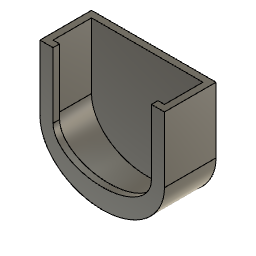
klarsteinHolder (Autodesk Fusion 360 design; units mm, degrees)
Autodesk Fusion 360 part; units mm, degrees
note: some values were not read from the file. Set by a fixed rule: which sketch regions a step uses.
sketch "out" plane through (0, 0, 0) normal (0, 1, 0) x (1, 0, 0)
  line L0 (0, 0) -> (57, 0)
  line L1 (57, 0) -> (57, -30)
  line L2 (57, -30) -> (0, -30)
  line L3 (0, -30) -> (0, 0)
  line L4 (0, 0) -> (57, 0) construction
  line L5 (57, 0) -> (57, 23) construction
  line L6 (57, 23) -> (0, 23) construction
  line L7 (0, 23) -> (0, 0) construction
  ellipse E0 centre (28.5, 0) end of major axis (57, 0) minor radius 23
  line L8 (0, 0) -> (57, 0)
  line L9 (28.5, -23) -> (28.5, 23)
  point P0 (28.5, 0)
  dimension "d25" = 57
  dimension "d26" = 30
  dimension "d27" = 57
  dimension "d28" = 23
  dimension "d29" = 46
  constraint horizontal L0
  constraint vertical L1
  constraint horizontal L2
  constraint vertical L3
  constraint horizontal L4
  constraint vertical L5
  constraint horizontal L6
  constraint vertical L7
  constraint coincident L0 P0
  constraint midpoint L4 P0
  constraint coincident P0 E0.centre
  constraint coincident L0.start E0
  constraint coincident L0.end E0
  constraint coincident E0 L9.start
  constraint coincident E0 L9.end
  measures "d25" distance of L0.start L0.end
  measures "d26" distance of L0.start L2.end
  measures "d27" distance of L0.start L0.end
  measures "d28" distance of L0.start L6.end
extrude "Extrude4" add sketch "out" along normal blind 23.6
ref_plane "WorkPlane2" through (0, 3, 0) normal (0, 1, 0) x (0, 0, 1)
sketch "inner" plane through (0, 3, 0) normal (0, 1, 0) x (1, 0, 0)
  line L0 (0, 0) -> (3, 0) construction
  line L1 (3, 0) -> (54, 0)
  line L2 (54, 0) -> (54, -50)
  line L3 (54, -50) -> (3, -50)
  line L4 (3, -50) -> (3, 0)
  line L5 (3, 0) -> (54, 0) construction
  line L6 (54, 0) -> (54, 20) construction
  line L7 (54, 20) -> (3, 20) construction
  line L8 (3, 20) -> (3, 0) construction
  ellipse E0 centre (28.5, 0) end of major axis (54, 0) minor radius 20
  line L9 (3, 0) -> (54, 0)
  line L10 (28.5, -20) -> (28.5, 20)
  point P0 (28.5, 0)
  dimension "d33" = 3
  dimension "d34" = 51
  dimension "d35" = 50
  dimension "d36" = 51
  dimension "d37" = 20
  constraint coincident L0.start origin
  constraint horizontal L0
  constraint horizontal L1
  constraint vertical L2
  constraint horizontal L3
  constraint vertical L4
  constraint horizontal L5
  constraint vertical L6
  constraint horizontal L7
  constraint vertical L8
  constraint coincident L1 P0
  constraint midpoint L1 P0
  constraint coincident L7 L10.end
  constraint midpoint L7 L10.end
  constraint coincident P0 E0.centre
  constraint coincident L0.end E0
  constraint coincident E0 L10.start
  measures "d33" distance of L0.start L0.end
  measures "d34" distance of L0.end L1.end
  measures "d35" distance of L0.end L3.end
  measures "d36" distance of L0.end L1.end
  measures "d37" distance of L0.end L7.end
extrude "Extrude5" cut sketch "inner" along normal blind 17.6
sketch "Sketch7" plane through (0, 0, 0) normal (0, 1, 0) x (1, 0, 0)
  line L0 (0, 0) -> (6, 0) construction
  line L1 (6, 0) -> (51, 0)
  line L2 (51, 0) -> (51, -50)
  line L3 (51, -50) -> (6, -50)
  line L4 (6, -50) -> (6, 0)
  line L5 (6, 0) -> (51, 0) construction
  line L6 (51, 0) -> (51, 14) construction
  line L7 (51, 14) -> (6, 14) construction
  line L8 (6, 14) -> (6, 0) construction
  ellipse E0 centre (28.5, 0) end of major axis (51, 0) minor radius 14
  line L9 (6, 0) -> (51, 0)
  line L10 (28.5, -14) -> (28.5, 14)
  point P0 (28.5, 0)
  dimension "d40" = 6
  dimension "d41" = 45
  dimension "d42" = 50
  dimension "d43" = 45
  dimension "d44" = 14
  constraint coincident L0.start origin
  constraint horizontal L0
  constraint horizontal L1
  constraint vertical L2
  constraint horizontal L3
  constraint vertical L4
  constraint horizontal L5
  constraint vertical L6
  constraint horizontal L7
  constraint vertical L8
  constraint coincident L1 P0
  constraint midpoint L5 P0
  constraint coincident L7 L10.end
  constraint midpoint L7 L10.end
  constraint coincident P0 E0.centre
  constraint coincident L0.end E0
  constraint coincident E0 L10.start
  measures "d40" distance of L0.start L0.end
  measures "d41" distance of L0.end L1.end
  measures "d42" distance of L0.end L3.end
  measures "d43" distance of L0.end L1.end
  measures "d44" distance of L0.end L7.end
extrude "Extrude6" cut sketch "Sketch7" along normal blind 3
equation "height = 50 mm"
equation "thickness = 3 mm"
equation "roundDiameter = 40 mm"
equation "inner = 17.6 mm"
equation "width = 51 mm"
equation "d25 = width + ( 2 * thickness )"
equation "d26 = height - ( roundDiameter / 2 )"
equation "d27 = width + ( 2 * thickness )"
equation "d28 = ( roundDiameter / 2 ) + thickness"
equation "d29 = roundDiameter + ( thickness * 2 )"
equation "d30 = inner + ( 2 * thickness )"
equation "d32 = thickness"
equation "d33 = thickness"
equation "d34 = width"
equation "d35 = height"
equation "d36 = width"
equation "d37 = roundDiameter / 2"
equation "d38 = inner"
equation "d40 = thickness * 2"
equation "d41 = width - ( 2 * thickness )"
equation "d42 = height"
equation "d43 = width - ( 2 * thickness )"
equation "d44 = roundDiameter / 2 - ( 2 * thickness )"
equation "d45 = thickness"
